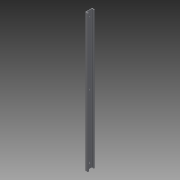
# Autodesk Inventor part: SAR340-40_b
Saved by Autodesk Inventor 2014 SP2 (Build 180246200, 246)
## iProperties
Created: 2019-05-01
Part Number: SAR340-40_b
Material: Generic
Catalog Web Link: www.cadenas.de
Description: SAR3_body-Slide Rails - Aluminum Alloy - Three - Step Slide Rails
Vendor: MISUMI
Document SubType Name: Modeling
Designer: psadmin
Manufacturer: MISUMI
Mass: 22.6226 g
Surface Area: 276.48 cm^2
Volume: 22.6226 cm^3
Density: 1 g/cm^3
Appearance: PSOLRGB-192-192-192
Category: PARTsolutions
Company: MISUMI
Title: SAR340-40
Author: Cadenas PARTsolutions
Comments: Slide Rails - Aluminum Alloy - Three - Step Slide Rails
PSOL_IDENT_0: {$CADENAS_DATA\23d-libs\misumi\metric\07_slide_rails\sar3_series\sar3_body.prj},167 {VTYP=3D},{NB=SA
PSOL_IDENT_1: R340-40_b},{LINA=SAR340-40},{NN=SAR3_body},{DATE=17.04.2019 06:32:12},{GEOMDATE=16.04.2019 09:38:26}
PSOL_IDENT_2: ,{VERSION=},{LINEID=10},{WBVAR=NO},{WBNUMERIC=NO}  {NB=SAR340-40_b},{LINA=SAR340-40},{KT=DUMMY},{PN=
PSOL_IDENT_3: SAR340-40},{TYPE=SAR340},{MAT1=Aluminum Alloy},{ST1=Clear Anodizing},{MAT2=Aluminum Alloy},{ST2=Clea
PSOL_IDENT_4: r Anodizing},{MAT3=Steel},{NO=40},{RL=400},{TD=460},{A=185},{B=370},{C=185},{D=370},{RLO=147},{BA=36
PSOL_IDENT_5: },{PPATH=sar3_series\\sar3_templ.prj}
NN: SAR3_body
NT: Slide Rails - Aluminum Alloy - Three - Step Slide Rails
NB: SAR340-40_b
NBSYN: $PN._b
LINA: SAR340-40
PN: SAR340-40
TYPE: SAR340
MAT1: Aluminum Alloy
ST1: Clear Anodizing
MAT2: Aluminum Alloy
ST2: Clear Anodizing
MAT3: Steel
NO: 40
RL: 400
TD: 460
RLO: 147
SUPPLIER: MISUMI
ARTICLENO: SAR340-40_b
BOMINFO: SAR340-40
CREATOR: CADENAS GmbH
Autodesk Inventor part; units mm, degrees
sketch "Sketch_1" plane through (0, 0, 0) normal (0, 0, 1) x (1, 0, 0)
  line L0 (-7.4, 19.7) -> (-7.4, 0.3)
  arc A0 (-7.4, 0.3) -> (-7.1, 0) centre (-7.1, 0.3) ccw
  line L1 (-7.1, 0) -> (-0.3, 0)
  arc A1 (-0.3, 0) -> (0, 0.3) centre (-0.3, 0.3) ccw
  line L2 (0, 0.3) -> (0, 2.95)
  arc A2 (0, 2.95) -> (-0.2, 3.15) centre (-0.2, 2.95) ccw
  line L3 (-0.2, 3.15) -> (-0.5141, 3.15)
  arc A3 (-0.5141, 3.15) -> (-0.708, 2.999) centre (-0.5141, 2.95) ccw
  arc A4 (-4.392, 2.999) -> (-0.708, 2.999) centre (-2.55, 3.465) ccw
  arc A5 (-4.392, 2.999) -> (-4.5859, 3.15) centre (-4.5859, 2.95) ccw
  line L4 (-4.5859, 3.15) -> (-5.8, 3.15)
  arc A6 (-6, 3.35) -> (-5.8, 3.15) centre (-5.8, 3.35) ccw
  line L5 (-6, 3.35) -> (-6, 16.65)
  arc A7 (-5.8, 16.85) -> (-6, 16.65) centre (-5.8, 16.65) ccw
  line L6 (-5.8, 16.85) -> (-4.5859, 16.85)
  arc A8 (-4.5859, 16.85) -> (-4.392, 17.001) centre (-4.5859, 17.05) ccw
  arc A9 (-0.708, 17.001) -> (-4.392, 17.001) centre (-2.55, 16.535) ccw
  arc A10 (-0.708, 17.001) -> (-0.5141, 16.85) centre (-0.5141, 17.05) ccw
  line L7 (-0.5141, 16.85) -> (-0.2, 16.85)
  arc A11 (-0.2, 16.85) -> (0, 17.05) centre (-0.2, 17.05) ccw
  line L8 (0, 17.05) -> (0, 19.7)
  arc A12 (0, 19.7) -> (-0.3, 20) centre (-0.3, 19.7) ccw
  line L9 (-0.3, 20) -> (-7.1, 20)
  arc A13 (-7.1, 20) -> (-7.4, 19.7) centre (-7.1, 19.7) ccw
  constraints: 28 point on circle, 20 end point, 14 centre point
extrude "Extrusion1" add sketch "Sketch_1" along normal blind 400
sketch "Sketch2" plane through (-6, 3.35, 0) normal (1, 0, 0) x (0, 0, -1)
  point P0 (-15, 6.65)
hole "Hole1" at (-6, 10, 15) direction (-1, 0, 0) diameter 3.5 depth 1.4 countersink diameter 6.1 countersink angle 90
pattern_linear "Rectangular Pattern1" count 3 spacing 185 along (0, 0, 1) of "Hole1"
ref_plane "to_rail_XY" through (0.6, 10, 200) normal (0, 0, 1) x (1, 0, 0)
ref_plane "to_rail_YZ" through (0.6, 10, 200) normal (1, 0, 0) x (0, 1, 0)
ref_plane "to_rail_ZX" through (0.6, 10, 200) normal (0, 1, 0) x (0, 0, 1)
body "Solid1"
